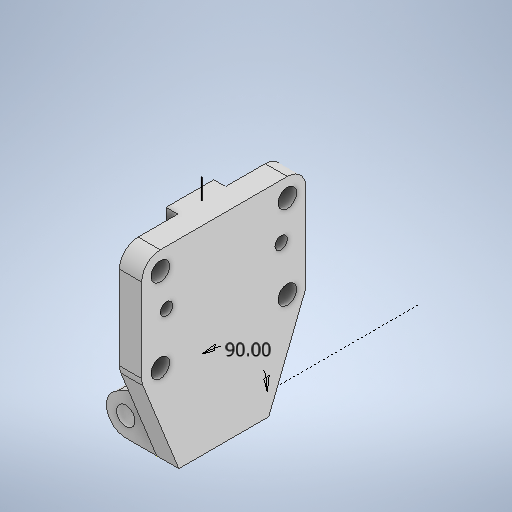
# Autodesk Inventor part: TheCamera
Saved by Autodesk Inventor 2025.1 (Build 291241000, 241)
## iProperties
Created: 2026-05-18
Part Number: TheCamera
Material: Generic
Document SubType Name: Modeling
Designer: User
Density: 1 g/cm^3
Appearance: Default
Author: User
## iProperties of the stored document TheCamera_3DPrint.ipt
Created: 2026-05-18
Part Number: TheCamera_3DPrint
Material: Generic
Document SubType Name: Modeling
Designer: User
Density: 1 g/cm^3
Appearance: Default
Author: User
Autodesk Inventor part; units mm, degrees
ref_plane "YZ Plane" through (0, 0, 0) normal (1, 0, 0) x (0, 1, 0)
sketch "Sketch1" plane through (0, 0, 0) normal (0, 0, 1) x (1, 0, 0)
  circle A0 centre (3, -3) radius 1.5 projected
  arc A1 (4.6242, -5.5223) -> (3, 0) centre (3, -3) ccw projected
  arc A2 (4.6783, -5.6064) -> (3, 0.1) centre (3, -3) ccw
  circle A3 centre (3, -3) radius 3.1
  point P0 (0, 0)
  point P1 (3, 0.1)
  dimension "d0" = 0.1
  constraints: 2 point on circle, 1 centre point, 1 coincident, 3 other
  measures "d0" radial gap between concentric circles of A1 A2
extrude "Extrusion1" add sketch "Sketch1" along normal blind 3.5
sketch "Sketch2" plane through (3, -3, 0) normal (0, 0, -1) x (-1, 0, 0)
  circle A0 centre (0, 0) radius 3.1 projected
  point P0 (3, 3)
extrude "Extrusion2" cut sketch "Sketch2" against normal blind 0.1
sketch "Sketch3" plane through (3, -3, 3.5) normal (0, 0, 1) x (1, 0, 0)
  circle A0 centre (0, 0) radius 3.1 projected
  line L0 (0, 3.1) -> (5, 3.1)
  line L1 (0, -3.1) -> (5, -3.1)
  line L2 (5, -3.1) -> (5, 3.1)
  point P0 (-3, 3)
  dimension "d5" = 5
  dimension "d6" = 5
  constraints: 6 end point, 2 horizontal, 2 point on circle, 2 tangent
  measures "d5" distance of L0.start L0.end
  measures "d6" distance of L1.start L1.end
ref_plane "Work Plane1" through (-0.6712, -8.5, -7.5) normal (0, 0, -1) x (0, 1, 0)
extrude "Extrusion3" add sketch "Sketch3" against normal up to surface (11 mm away) contours A0 L0 L2 L1
sketch "Sketch4" plane through (8, 0.1, -7.5) normal (0, 0, -1) x (-1, 0, 0)
  arc A0 (5, 0) -> (5, -6.2) centre (5, -3.1) ccw projected
  line L0 (0, 0) -> (5, 0) projected
  line L1 (0, -6.2) -> (0, 0) projected
  line L2 (5, -6.2) -> (0, -6.2) projected
  point P0 (8, -0.1)
extrude "Extrusion4" add sketch "Sketch4" along normal blind 0.1
sketch "Sketch5" plane through (8, 0.1, -7.6) normal (0, 0, -1) x (-1, 0, 0)
  arc A0 (5, -6.2) -> (5, 0) centre (5, -3.1) ccw projected
  line L0 (5, -6.2) -> (0, -6.2) projected
  line L1 (0, -6.2) -> (0, 0) projected
  line L2 (0, 0) -> (5, 0) projected
  circle A1 centre (5, -3.1) radius 1.5 projected
  point P0 (8, -0.1)
extrude "Extrusion5" add sketch "Sketch5" along normal blind 3.4
sketch "Sketch6" plane through (3, 0.1, 3.5) normal (0, 1, 0) x (1, 0, 0)
  line L0 (0, 3.5) -> (3, 3.5) projected
  line L1 (0, 11.1) -> (3.1, 11.1) projected
  line L2 (0, 3.4) -> (0, 11.1) projected
  line L3 (0, 3.4) -> (3.1, 3.4) projected
  line L4 (3.1, 3.4) -> (0, 3.4)
  line L5 (0, 3.4) -> (0, 11.1)
  line L6 (0, 11.1) -> (3.1, 11.1)
  line L7 (3.1, 11.1) -> (3.1, 3.4)
  point P0 (-3, 3.5)
  constraints: 8 end point, 2 parallel, 1 horizontal, 1 perpendicular
extrude "Extrusion6" cut sketch "Sketch6" against normal through all
sketch "Sketch7" plane through (8, -6.1, 3.5) normal (1, 0, 0) x (0, 0, -1)
  line L0 (0, 0) -> (14.5, 0) projected
  line L1 (7.25, 0) -> (7.25, 35.3128)
  line L2 (7.25, 0) -> (42.5628, 0) construction
  point P0 (3.5, 6.1)
  dimension "d15" = 90
  constraints: 4 end point, 1 horizontal, 1 midpoint, 1 perpendicular
  measures "d15" angle of L2 L1
sketch "Sketch8" plane through (8, -6.1, 3.5) normal (1, 0, 0) x (0, 0, -1)
  circle A0 centre (-3.0004, 15.5784) radius 1.1 projected
  circle A1 centre (-3.0004, 29.0784) radius 1.1 projected
  circle A2 centre (17.4996, 29.0784) radius 1.1 projected
  circle A3 centre (17.4996, 15.5784) radius 1.1 projected
  circle A4 centre (-3.0004, 15.5784) radius 1.5
  circle A5 centre (-3.0004, 29.0784) radius 1.5
  circle A6 centre (17.4996, 29.0784) radius 1.5
  circle A7 centre (17.4996, 15.5784) radius 1.5
  circle A8 centre (17.4996, 15.5784) radius 3
  circle A9 centre (17.4996, 29.0784) radius 3
  circle A10 centre (-3.0004, 29.0784) radius 3
  circle A11 centre (-3.0004, 15.5784) radius 3
  line L0 (-3.0004, 32.0784) -> (17.4996, 32.0784)
  line L1 (-6.0004, 29.0784) -> (-6.0004, 15.5784)
  line L2 (20.4996, 29.0784) -> (20.4996, 15.5784)
  line L3 (-3.0004, 12.5784) -> (17.4996, 12.5784)
  line L4 (0, 6.2) -> (14.5, 6.2) projected
  line L5 (0, 0) -> (0, 6.2) projected
  line L6 (0, 0) -> (14.5, 0) projected
  line L7 (14.5, 6.2) -> (14.5, 0) projected
  line L8 (0, 0) -> (-5.7858, 14.4642)
  line L9 (14.5, 0) -> (20.2851, 14.4643)
  point P0 (3.5, 6.1)
  dimension "d16" = 3
  dimension "d17" = 3
  dimension "d18" = 3
  dimension "d19" = 3
  dimension "d20" = 6
  dimension "d21" = 6
  dimension "d22" = 6
  dimension "d23" = 6
  constraints: 12 end point, 10 point on circle, 8 centre point, 8 coincident, 7 tangent, 1 perpendicular
  measures "d16" diameter of A4
  measures "d17" diameter of A5
  measures "d18" diameter of A6
  measures "d19" diameter of A7
  measures "d20" diameter of A8
  measures "d21" diameter of A9
  measures "d22" diameter of A10
  measures "d23" diameter of A11
ref_plane "Work Plane2" through (11.5705, 1.2284, -16.2496) normal (-1, 0, 0) x (0, 0, 1)
extrude "Extrusion7" add sketch "Sketch8" along normal up to surface (3.5705 mm away) contours A8 | A8 L3 A11 L1 A10 L0 A9 L2 | A8 L9 L7 L4 L5 L8 A11 L3 | A9 | A11 | L6 L5 L4 L7 | A10
sketch "Sketch9" plane through (3, 0.1, 3.5) normal (0, 1, 0) x (1, 0, 0)
  line L0 (3.1, 11.1) -> (3.1, 3.4) projected
  line L1 (5, 17.4996) -> (5, -3.0004) projected
  line L2 (3.1, 11.1) -> (0, 11.1) projected
  line L3 (3.1, 11.1) -> (5, 11.1)
  line L4 (5, 11.1) -> (5, 3.4)
  line L5 (5, 3.4) -> (3.1, 3.4)
  line L6 (3.1, 3.4) -> (3.1, 11.1)
  point P0 (-3, 3.5)
  point P1 (3.1, 3.4)
  point P2 (5, 11.1)
  constraints: 8 end point, 2 parallel, 1 horizontal, 1 perpendicular, 1 point on line
extrude "Extrusion8" add sketch "Sketch9" along normal up to surface (25.8784 mm away)
sketch "Sketch10" plane through (11.5705, 9.4784, -16.9996) normal (1, 0, 0) x (0, 0, -1)
  circle A0 centre (-22.5, 7.75) radius 0.5 projected
  circle A1 centre (-4, 7.75) radius 0.5 projected
  circle A2 centre (-22.5, 7.75) radius 1
  circle A3 centre (-4, 7.75) radius 1
  point P0 (-16.9996, -9.4784)
  dimension "d29" = 2
  dimension "d30" = 2
  constraints: 2 centre point, 2 coincident
  measures "d29" diameter of A2
  measures "d30" diameter of A3
extrude "Extrusion9" cut sketch "Sketch10" against normal through all contours A0 | A1 | A2 | A3
chamfer "Chamfer1" distance 5 angle 45 2 edges at (8, 0.1, 1.8) (8, 0.1, -9.3)
fillet "Fillet1" radius 13 2 edges at (3, 0.1, -9.3) (3, 0.1, 1.8)
body "Solid1"
